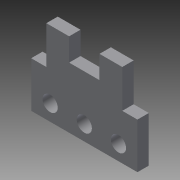
# Autodesk Inventor part: P1-6
Saved by Autodesk Inventor 2014 (Build 180170000, 170)
## iProperties
Created: 2017-02-06
Part Number: P1-6
Material: Generic
Document SubType Name: Modeling
Designer: mschaffel
Density: 1 g/cm^3
Appearance: Default
Author: mschaffel
Autodesk Inventor part; units mm, degrees
ref_plane "YZ Plane" through (0, 0, 0) normal (1, 0, 0) x (0, 1, 0)
ref_plane "XZ Plane" through (0, 0, 0) normal (0, 1, 0) x (-1, 0, 0)
ref_plane "XY Plane" through (0, 0, 0) normal (0, 0, 1) x (1, 0, 0)
sketch "Sketch1" plane through (0, 0, 0) normal (0, 1, 0) x (-1, 0, 0)
  line L0 (0, 0) -> (0, 60)
  line L1 (0, 60) -> (20, 60)
  line L2 (20, 60) -> (20, 110)
  line L3 (20, 110) -> (50, 110)
  line L4 (50, 110) -> (50, 80)
  line L5 (50, 80) -> (90, 80)
  line L6 (90, 80) -> (90, 110)
  line L7 (90, 110) -> (120, 110)
  line L8 (120, 110) -> (120, 60)
  line L9 (120, 60) -> (140, 60)
  line L10 (140, 60) -> (140, 0)
  line L11 (140, 0) -> (0, 0)
  circle A0 centre (25, 20) radius 10
  circle A1 centre (70, 20) radius 10
  circle A2 centre (115, 21) radius 10
  dimension "d0" = 50
  dimension "d1" = 20
  dimension "d2" = 20
  dimension "d5" = 20
  constraints: 24 end point, 8 parallel, 3 centre point, 1 collinear, 1 perpendicular, 1 vertical
  measures "d0" distance of L1.end L2.end
  measures "d1" diameter of A0
  measures "d2" diameter of A1
  measures "d5" diameter of A2
extrude "Extrusion1" add sketch "Sketch1" along normal blind 15
body "Solid1"
